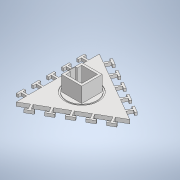
# Autodesk Inventor part: Base
Saved by Autodesk Inventor 2022.3 (Build 263350000, 350)
## iProperties
Created: 2023-03-28
Part Number: Base
Material: Generic
Document SubType Name: Modeling
Designer: Manuel Hueso Béjar
Density: 1 g/cm^3
Appearance: Default
Author: Manuel Hueso Béjar
Autodesk Inventor part; units mm, degrees
ref_plane "YZ Plane" through (0, 0, 0) normal (1, 0, 0) x (0, 1, 0)
ref_plane "XZ Plane" through (0, 0, 0) normal (0, 1, 0) x (-1, 0, 0)
ref_plane "XY Plane" through (0, 0, 0) normal (0, 0, 1) x (1, 0, 0)
sketch "Sketch1" plane through (0, 0, 0) normal (0, 1, 0) x (-1, 0, 0)
  circle A0 centre (0, 0) radius 127.0171
  line L0 (-127.0171, 220) -> (254.0341, 0)
  line L1 (254.0341, 0) -> (-127.0171, -220)
  line L2 (-127.0171, -220) -> (-127.0171, 220)
  line L3 (63.5085, 110) -> (63.5085, -110)
  line L4 (63.5085, 110) -> (-127.0171, 0)
  line L5 (-127.0171, 0) -> (63.5085, -110)
  line L6 (46.0085, 2.5) -> (81.0085, 2.5)
  line L7 (81.0085, 2.5) -> (81.0085, -2.5)
  line L8 (81.0085, -2.5) -> (46.0085, -2.5)
  line L9 (46.0085, -2.5) -> (46.0085, 2.5)
  line L10 (46.0085, 2.5) -> (81.0085, -2.5) construction
  line L11 (81.0085, 2.5) -> (46.0085, -2.5) construction
  line L12 (78.5085, 10) -> (83.5085, 10)
  line L13 (83.5085, 10) -> (83.5085, -10)
  line L14 (83.5085, -10) -> (78.5085, -10)
  line L15 (78.5085, -10) -> (78.5085, 10)
  line L16 (78.5085, 10) -> (83.5085, -10) construction
  line L17 (83.5085, 10) -> (78.5085, -10) construction
  line L18 (78.5085, 30) -> (78.5085, 50)
  line L19 (78.5085, 50) -> (83.5085, 50)
  line L20 (83.5085, 50) -> (83.5085, 30)
  line L21 (83.5085, 30) -> (78.5085, 30)
  line L22 (46.0085, 42.5) -> (81.0085, 42.5)
  line L23 (81.0085, 37.5) -> (46.0085, 37.5)
  line L24 (78.5085, 70) -> (78.5085, 90)
  line L25 (78.5085, 90) -> (83.5085, 90)
  line L26 (83.5085, 90) -> (83.5085, 70)
  line L27 (83.5085, 70) -> (78.5085, 70)
  line L28 (46.0085, 82.5) -> (81.0085, 82.5)
  line L29 (81.0085, 77.5) -> (46.0085, 77.5)
  line L30 (78.5085, -50) -> (78.5085, -30)
  line L31 (78.5085, -30) -> (83.5085, -30)
  line L32 (83.5085, -30) -> (83.5085, -50)
  line L33 (83.5085, -50) -> (78.5085, -50)
  line L34 (46.0085, -37.5) -> (81.0085, -37.5)
  line L35 (81.0085, -42.5) -> (46.0085, -42.5)
  line L36 (78.5085, -10) -> (78.5085, 10)
  line L37 (78.5085, 10) -> (83.5085, 10)
  line L38 (83.5085, 10) -> (83.5085, -10)
  line L39 (83.5085, -10) -> (78.5085, -10)
  line L40 (46.0085, 2.5) -> (81.0085, 2.5)
  line L41 (81.0085, -2.5) -> (46.0085, -2.5)
  line L42 (78.5085, 30) -> (78.5085, 50)
  line L43 (78.5085, 50) -> (83.5085, 50)
  line L44 (83.5085, 50) -> (83.5085, 30)
  line L45 (83.5085, 30) -> (78.5085, 30)
  line L46 (46.0085, 42.5) -> (81.0085, 42.5)
  line L47 (81.0085, 37.5) -> (46.0085, 37.5)
  line L48 (78.5085, -90) -> (78.5085, -70)
  line L49 (78.5085, -70) -> (83.5085, -70)
  line L50 (83.5085, -70) -> (83.5085, -90)
  line L51 (83.5085, -90) -> (78.5085, -90)
  line L52 (46.0085, -77.5) -> (81.0085, -77.5)
  line L53 (81.0085, -82.5) -> (46.0085, -82.5)
  line L54 (78.5085, -50) -> (78.5085, -30)
  line L55 (78.5085, -30) -> (83.5085, -30)
  line L56 (83.5085, -30) -> (83.5085, -50)
  line L57 (83.5085, -50) -> (78.5085, -50)
  line L58 (46.0085, -37.5) -> (81.0085, -37.5)
  line L59 (81.0085, -42.5) -> (46.0085, -42.5)
  line L60 (78.5085, -10) -> (78.5085, 10)
  line L61 (78.5085, 10) -> (83.5085, 10)
  line L62 (83.5085, 10) -> (83.5085, -10)
  line L63 (83.5085, -10) -> (78.5085, -10)
  line L64 (46.0085, 2.5) -> (81.0085, 2.5)
  line L65 (81.0085, -2.5) -> (46.0085, -2.5)
  line L66 (-25.1693, 38.5946) -> (-42.6693, 68.9054)
  line L67 (-30.594, 72.9904) -> (-47.9145, 62.9904)
  line L68 (-47.9145, 62.9904) -> (-50.4145, 67.3205)
  line L69 (-50.4145, 67.3205) -> (-33.094, 77.3205)
  line L70 (-33.094, 77.3205) -> (-30.594, 72.9904)
  line L71 (-38.3392, 71.4054) -> (-20.8392, 41.0946)
  line L72 (-20.8392, -41.0946) -> (-38.3392, -71.4054)
  line L73 (-47.9145, -62.9904) -> (-30.594, -72.9904)
  line L74 (-30.594, -72.9904) -> (-33.094, -77.3205)
  line L75 (-33.094, -77.3205) -> (-50.4145, -67.3205)
  line L76 (-50.4145, -67.3205) -> (-47.9145, -62.9904)
  line L77 (-42.6693, -68.9054) -> (-25.1693, -38.5946)
  line L78 (-85.0555, 47.3205) -> (-67.735, 57.3205)
  line L79 (-67.735, 57.3205) -> (-65.235, 52.9904)
  line L80 (-65.235, 52.9904) -> (-82.5555, 42.9904)
  line L81 (-72.9802, 51.4054) -> (-55.4802, 21.0946)
  line L82 (-59.8103, 18.5946) -> (-77.3103, 48.9054)
  line L83 (-82.5555, 42.9904) -> (-85.0555, 47.3205)
  line L84 (-119.6966, 27.3205) -> (-102.376, 37.3205)
  line L85 (-102.376, 37.3205) -> (-99.876, 32.9904)
  line L86 (-99.876, 32.9904) -> (-117.1966, 22.9904)
  line L87 (-107.6212, 31.4054) -> (-90.1212, 1.0946)
  line L88 (-94.4514, -1.4054) -> (-111.9514, 28.9054)
  line L89 (-117.1966, 22.9904) -> (-119.6966, 27.3205)
  line L90 (-15.7735, 87.3205) -> (1.547, 97.3205)
  line L91 (1.547, 97.3205) -> (4.047, 92.9904)
  line L92 (4.047, 92.9904) -> (-13.2735, 82.9904)
  line L93 (-3.6982, 91.4054) -> (13.8018, 61.0946)
  line L94 (9.4717, 58.5946) -> (-8.0283, 88.9054)
  line L95 (-13.2735, 82.9904) -> (-15.7735, 87.3205)
  line L96 (-50.4145, 67.3205) -> (-33.094, 77.3205)
  line L97 (-33.094, 77.3205) -> (-30.594, 72.9904)
  line L98 (-30.594, 72.9904) -> (-47.9145, 62.9904)
  line L99 (-38.3392, 71.4054) -> (-20.8392, 41.0946)
  line L100 (-25.1693, 38.5946) -> (-42.6693, 68.9054)
  line L101 (-47.9145, 62.9904) -> (-50.4145, 67.3205)
  line L102 (-85.0555, 47.3205) -> (-67.735, 57.3205)
  line L103 (-67.735, 57.3205) -> (-65.235, 52.9904)
  line L104 (-65.235, 52.9904) -> (-82.5555, 42.9904)
  line L105 (-72.9802, 51.4054) -> (-55.4802, 21.0946)
  line L106 (-59.8103, 18.5946) -> (-77.3103, 48.9054)
  line L107 (-82.5555, 42.9904) -> (-85.0555, 47.3205)
  line L108 (18.8675, 107.3205) -> (36.188, 117.3205)
  line L109 (36.188, 117.3205) -> (38.688, 112.9904)
  line L110 (38.688, 112.9904) -> (21.3675, 102.9904)
  line L111 (30.9428, 111.4054) -> (48.4428, 81.0946)
  line L112 (44.1127, 78.5946) -> (26.6127, 108.9054)
  line L113 (21.3675, 102.9904) -> (18.8675, 107.3205)
  line L114 (-15.7735, 87.3205) -> (1.547, 97.3205)
  line L115 (1.547, 97.3205) -> (4.047, 92.9904)
  line L116 (4.047, 92.9904) -> (-13.2735, 82.9904)
  line L117 (-3.6982, 91.4054) -> (13.8018, 61.0946)
  line L118 (9.4717, 58.5946) -> (-8.0283, 88.9054)
  line L119 (-13.2735, 82.9904) -> (-15.7735, 87.3205)
  line L120 (-50.4145, 67.3205) -> (-33.094, 77.3205)
  line L121 (-33.094, 77.3205) -> (-30.594, 72.9904)
  line L122 (-30.594, 72.9904) -> (-47.9145, 62.9904)
  line L123 (-38.3392, 71.4054) -> (-20.8392, 41.0946)
  line L124 (-25.1693, 38.5946) -> (-42.6693, 68.9054)
  line L125 (-47.9145, 62.9904) -> (-50.4145, 67.3205)
  line L126 (-77.3103, -48.9054) -> (-59.8103, -18.5946)
  line L127 (-82.5555, -42.9904) -> (-65.235, -52.9904)
  line L128 (-85.0555, -47.3205) -> (-82.5555, -42.9904)
  line L129 (-67.735, -57.3205) -> (-85.0555, -47.3205)
  line L130 (-65.235, -52.9904) -> (-67.735, -57.3205)
  line L131 (-55.4802, -21.0946) -> (-72.9802, -51.4054)
  line L132 (-111.9514, -28.9054) -> (-94.4514, 1.4054)
  line L133 (-117.1966, -22.9904) -> (-99.876, -32.9904)
  line L134 (-119.6966, -27.3205) -> (-117.1966, -22.9904)
  line L135 (-102.376, -37.3205) -> (-119.6966, -27.3205)
  line L136 (-99.876, -32.9904) -> (-102.376, -37.3205)
  line L137 (-90.1212, -1.0946) -> (-107.6212, -31.4054)
  line L138 (-8.0283, -88.9054) -> (9.4717, -58.5946)
  line L139 (-13.2735, -82.9904) -> (4.047, -92.9904)
  line L140 (-15.7735, -87.3205) -> (-13.2735, -82.9904)
  line L141 (1.547, -97.3205) -> (-15.7735, -87.3205)
  line L142 (4.047, -92.9904) -> (1.547, -97.3205)
  line L143 (13.8018, -61.0946) -> (-3.6982, -91.4054)
  line L144 (-42.6693, -68.9054) -> (-25.1693, -38.5946)
  line L145 (-47.9145, -62.9904) -> (-30.594, -72.9904)
  line L146 (-50.4145, -67.3205) -> (-47.9145, -62.9904)
  line L147 (-33.094, -77.3205) -> (-50.4145, -67.3205)
  line L148 (-30.594, -72.9904) -> (-33.094, -77.3205)
  line L149 (-20.8392, -41.0946) -> (-38.3392, -71.4054)
  line L150 (-77.3103, -48.9054) -> (-59.8103, -18.5946)
  line L151 (-82.5555, -42.9904) -> (-65.235, -52.9904)
  line L152 (-85.0555, -47.3205) -> (-82.5555, -42.9904)
  line L153 (-67.735, -57.3205) -> (-85.0555, -47.3205)
  line L154 (-65.235, -52.9904) -> (-67.735, -57.3205)
  line L155 (-55.4802, -21.0946) -> (-72.9802, -51.4054)
  line L156 (26.6127, -108.9054) -> (44.1127, -78.5946)
  line L157 (21.3675, -102.9904) -> (38.688, -112.9904)
  line L158 (18.8675, -107.3205) -> (21.3675, -102.9904)
  line L159 (36.188, -117.3205) -> (18.8675, -107.3205)
  line L160 (38.688, -112.9904) -> (36.188, -117.3205)
  line L161 (48.4428, -81.0946) -> (30.9428, -111.4054)
  line L162 (-8.0283, -88.9054) -> (9.4717, -58.5946)
  line L163 (-13.2735, -82.9904) -> (4.047, -92.9904)
  line L164 (-15.7735, -87.3205) -> (-13.2735, -82.9904)
  line L165 (1.547, -97.3205) -> (-15.7735, -87.3205)
  line L166 (4.047, -92.9904) -> (1.547, -97.3205)
  line L167 (13.8018, -61.0946) -> (-3.6982, -91.4054)
  line L168 (-42.6693, -68.9054) -> (-25.1693, -38.5946)
  line L169 (-47.9145, -62.9904) -> (-30.594, -72.9904)
  line L170 (-50.4145, -67.3205) -> (-47.9145, -62.9904)
  line L171 (-33.094, -77.3205) -> (-50.4145, -67.3205)
  line L172 (-30.594, -72.9904) -> (-33.094, -77.3205)
  line L173 (-20.8392, -41.0946) -> (-38.3392, -71.4054)
  point P0 (63.5085, 0)
  point P1 (81.0085, 0)
  point P2 (78.5085, -2.5)
  point P3 (78.5085, 2.5)
  point P4 (63.5085, 2.5)
  point P5 (63.5085, 37.5)
  point P6 (78.5085, 37.5)
  point P7 (78.5085, 42.5)
  point P8 (63.5085, 42.5)
  point P9 (63.5085, 77.5)
  point P10 (78.5085, 77.5)
  point P11 (78.5085, 82.5)
  point P12 (63.5085, 82.5)
  point P13 (39.6928, 96.25)
  point P14 (32.1928, 109.2404)
  point P15 (27.8627, 106.7404)
  point P16 (35.3627, 93.75)
  point P17 (5.0518, 76.25)
  point P18 (-2.4482, 89.2404)
  point P19 (-6.7783, 86.7404)
  point P20 (0.7217, 73.75)
  point P21 (-29.5892, 56.25)
  point P22 (-37.0892, 69.2404)
  point P23 (-41.4193, 66.7404)
  point P24 (-33.9193, 53.75)
  point P25 (-64.2302, 36.25)
  point P26 (-71.7302, 49.2404)
  point P27 (-76.0603, 46.7404)
  point P28 (-68.5603, 33.75)
  point P29 (-98.8712, 16.25)
  point P30 (-106.3712, 29.2404)
  point P31 (-110.7014, 26.7404)
  point P32 (-103.2014, 13.75)
  point P33 (-103.2014, -13.75)
  point P34 (-110.7014, -26.7404)
  point P35 (-106.3712, -29.2404)
  point P36 (-98.8712, -16.25)
  point P37 (-68.5603, -33.75)
  point P38 (-76.0603, -46.7404)
  point P39 (-71.7302, -49.2404)
  point P40 (-64.2302, -36.25)
  point P41 (-33.9193, -53.75)
  point P42 (-41.4193, -66.7404)
  point P43 (-37.0892, -69.2404)
  point P44 (-29.5892, -56.25)
  point P45 (0.7217, -73.75)
  point P46 (-6.7783, -86.7404)
  point P47 (-2.4482, -89.2404)
  point P48 (5.0518, -76.25)
  point P49 (35.3627, -93.75)
  point P50 (27.8627, -106.7404)
  point P51 (32.1928, -109.2404)
  point P52 (39.6928, -96.25)
  point P53 (63.5085, -82.5)
  point P54 (78.5085, -82.5)
  point P55 (78.5085, -77.5)
  point P56 (63.5085, -77.5)
  point P57 (63.5085, -42.5)
  point P58 (78.5085, -42.5)
  point P59 (78.5085, -37.5)
  point P60 (63.5085, -37.5)
  point P61 (63.5085, -2.5)
  dimension "d1" = 220
  dimension "d2" = 35
  dimension "d3" = 5
  dimension "d4" = 5
  dimension "d5" = 20
  dimension "d8" = 40
  dimension "d11" = 40
  dimension "d16" = 240
  dimension "d20" = 40
  dimension "d23" = 40
  dimension "d28" = 40
  dimension "d31" = 40
  constraints: 348 end point, 9 midpoint, 4 parallel, 2 coincident, 2 horizontal, 2 perpendicular, 2 vertical, 1 horizontal alignment, 378 other
  measures "d1" distance of L3.start L3.end
  measures "d2" distance of L7.end L8.end
  measures "d3" distance of L6.end L7.end
  measures "d4" distance of L13.end L14.end
  measures "d5" distance of L12.end L13.end
  measures "d8" distance of L14.end L18.start
  measures "d11" distance of L14.end L30.start
  measures "d20" distance of L68.end L78.start
  measures "d23" distance of L68.end L90.start
  measures "d28" distance of L77.start L126.start
  measures "d31" distance of L77.start L138.start
extrude "Extrusion1" add sketch "Sketch1" along normal blind 10 contours L3 L28 L111 L4 | L5 L161 L53 L3 | L4 L88 L132 L5 | L28 L24 L29 L3 | L3 L6 L9 L8 L53 L161 L5 L132 L88 L4 L111 L28 | L4 L112 L110 L111 | L3 L52 L48 L53 | L161 L157 L156 L5 | L88 L86 L87 L4 | L5 L137 L133 L132 | L24 L25 L26 L27 | L110 L113 L108 L109 | L48 L49 L50 L51 | L157 L160 L159 L158 | L86 L89 L84 L85 | L133 L136 L135 L134 | L22 L18 L23 L3 | L4 L94 L92 L93 | L3 L34 L30 L35 | L143 L139 L138 L5 | L82 L80 L81 L4 | L5 L131 L127 L126 | L18 L19 L20 L21 | L92 L95 L90 L91 | L30 L31 L32 L33 | L139 L142 L141 L140 | L80 L83 L78 L79 | L127 L130 L129 L128 | L6 L15 L8 L3 | L3 L8 L9 L6 | L4 L66 L67 L71 | L72 L73 L77 L5 | L15 L12 L13 L14 L8 L7 L6 | L6 L7 L8 L15 | L67 L68 L69 L70 | L73 L74 L75 L76
extrude "Extrusion2" cut sketch "Sketch1" along normal blind 2.5 contours L28 L24 L29 L3 | L4 L112 L110 L111 | L3 L52 L48 L53 | L161 L157 L156 L5 | L88 L86 L87 L4 | L5 L137 L133 L132 | L24 L25 L26 L27 | L110 L113 L108 L109 | L48 L49 L50 L51 | L157 L160 L159 L158 | L86 L89 L84 L85 | L133 L136 L135 L134 | L22 L18 L23 L3 | L4 L94 L92 L93 | L3 L34 L30 L35 | L143 L139 L138 L5 | L82 L80 L81 L4 | L5 L131 L127 L126 | L18 L19 L20 L21 | L92 L95 L90 L91 | L30 L31 L32 L33 | L139 L142 L141 L140 | L80 L83 L78 L79 | L127 L130 L129 L128 | L6 L15 L8 L3 | L4 L66 L67 L71 | L72 L73 L77 L5 | L15 L12 L13 L14 L8 L7 L6 | L6 L7 L8 L15 | L67 L68 L69 L70 | L73 L74 L75 L76
sketch "Sketch2" plane through (0, 10, 0) normal (0, 1, 0) x (1, 0, 0)
  line L0 (-63.5085, 110) -> (-63.5085, -110) projected
  line L1 (-63.5085, 110) -> (31.7543, -55)
  line L2 (-63.5085, -110) -> (127.0171, 0) projected
  line L3 (127.0171, 0) -> (-63.5085, 0)
  line L4 (-63.5085, 110) -> (-63.5085, -110) projected
  line L5 (-63.5085, -110) -> (31.7543, 55)
  line L6 (127.0171, 0) -> (-63.5085, 110) projected
  line L7 (21, -21) -> (-21, -21)
  line L8 (-21, -21) -> (-21, 21)
  line L9 (-21, 21) -> (21, 21)
  line L10 (21, 21) -> (21, -21)
  line L11 (21, -21) -> (-21, 21) construction
  line L12 (-21, -21) -> (21, 21) construction
  line L13 (-27, 27) -> (-27, -27)
  line L14 (-27, -27) -> (27, -27)
  line L15 (27, -27) -> (27, 27)
  line L16 (27, 27) -> (-27, 27)
  line L17 (-26, 9) -> (-16, 9)
  line L18 (-16, 9) -> (-16, -9)
  line L19 (-16, -9) -> (-26, -9)
  line L20 (-26, -9) -> (-26, 9)
  line L21 (-26, 9) -> (-16, -9) construction
  line L22 (-16, 9) -> (-26, -9) construction
  point P0 (0, 0)
  point P1 (-63.5085, 82.5)
  point P2 (-0.7217, -73.75)
  point P3 (29.5892, -56.25)
  point P4 (-63.5085, -82.5)
  point P5 (-21, 0)
  point P6 (-21, -9)
  point P7 (-21, 9)
  point P8 (-63.5085, -2.5)
  dimension "d38" = 42
  dimension "d39" = 42
  dimension "d40" = 6
  dimension "d42" = 10
  dimension "d43" = 18
  constraints: 38 end point, 6 midpoint, 6 parallel, 4 perpendicular, 3 horizontal, 3 other
  measures "d38" distance of L8.end L9.end
  measures "d39" distance of L7.end L8.end
  measures "d40" distance between parallel lines of L8 L13
  measures "d42" distance of L18.end L19.end
  measures "d43" distance of L17.end L18.end
extrude "Extrusion3" add sketch "Sketch2" along normal blind 40 contours L16 L5 L9 L1 | L1 L9 L8 L17 L20 L3 L13 L16 | L3 L20 L19 L8 L7 L5 L14 L13 | L16 L15 L3 L10 L9 L5 | L5 L7 L1 L14 | L15 L14 L1 L7 L10 L3
sketch "Sketch3" plane through (0, 0, 0) normal (0, -1, 0) x (1, 0, 0)
  circle A0 centre (0, 0) radius 63.5085
  line L0 (-63.5085, -110) -> (-63.5085, 110) projected
  line L1 (-63.5085, 110) -> (127.0171, 0)
  line L2 (127.0171, 0) -> (-63.5085, -110)
  line L3 (-63.5085, -110) -> (-63.5085, 110)
  line L4 (-43.5085, -75.359) -> (87.0171, 0)
  line L5 (87.0171, 0) -> (-43.5085, 75.359)
  line L6 (-43.5085, 75.359) -> (-43.5085, -75.359)
  line L7 (-38.5085, -66.6987) -> (77.0171, 0)
  line L8 (77.0171, 0) -> (-38.5085, 66.6987)
  line L9 (-38.5085, 66.6987) -> (-38.5085, -66.6987)
  point P0 (-63.5085, 0)
  dimension "d41" = 20
  dimension "d46" = 5
  constraints: 18 end point, 2 coincident, 2 midpoint, 1 centre point, 11 other
  measures "d41" distance between parallel lines of L2 L4
  measures "d46" distance between parallel lines of L6 L9
extrude "Extrusion4" cut sketch "Sketch3" against normal blind 3 contours L8 A0 L5 | A0 L5 L4 L7 L8 | A0 L4 L7 | L8 L9 A0 L6 L5 | A0 L4 L6 L9 L7 | L9 A0 L6
sketch "Sketch4" plane through (-27, 10, -27) normal (-1, 0, 0) x (0, 0, 1)
  line L0 (18, 0) -> (18, 40) projected
  line L1 (36, 0) -> (36, 40) projected
  line L2 (18, 0) -> (36, 0)
  line L3 (36, 0) -> (36, 10)
  line L4 (36, 10) -> (18, 10)
  line L5 (18, 10) -> (18, 0)
  point P0 (27, -10)
  point P1 (18, 10)
  dimension "d49" = 10
  constraints: 8 end point, 2 parallel, 1 horizontal, 1 perpendicular, 1 point on line
  measures "d49" distance of L3.end L2.end
extrude "Extrusion5" cut sketch "Sketch4" against normal up to surface (1 mm away)
sketch "Sketch5" plane through (0, 10, 0) normal (0, 1, 0) x (1, 0, 0)
  circle A0 centre (0, 0) radius 40
  circle A1 centre (0, 0) radius 44
  dimension "d52" = 80
  dimension "d53" = 4
  constraints: 2 centre point, 1 coincident
  measures "d52" diameter of A0
  measures "d53" radial gap between concentric circles of A0 A1
extrude "Extrusion6" cut sketch "Sketch5" against normal blind 2
body "Solid1"
